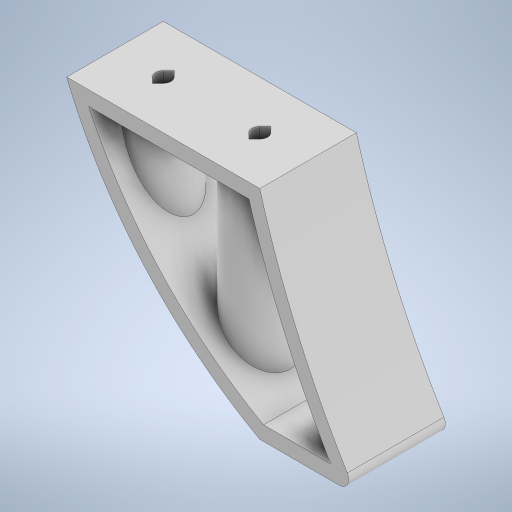
# Autodesk Inventor part: Feet
Saved by Autodesk Inventor 2023.1 (Build 271208000, 208)
## iProperties
Created: 2022-11-07
Part Number: Feet
Material: Generic
Document SubType Name: Modeling
Designer: nicol
Density: 1 g/cm^3
Appearance: Default
Author: nicol
Autodesk Inventor part; units mm, degrees
ref_plane "YZ Plane" through (0, 0, 0) normal (1, 0, 0) x (0, 1, 0)
ref_plane "XZ Plane" through (0, 0, 0) normal (0, 1, 0) x (-1, 0, 0)
ref_plane "XY Plane" through (0, 0, 0) normal (0, 0, 1) x (1, 0, 0)
sketch "Sketch1" plane through (0, 0, 0) normal (0, 0, 1) x (1, 0, 0)
  line L0 (0, 0) -> (20, 0)
  line L1 (-40, 45) -> (0, 45)
  arc A0 (-40, 45) -> (0, 0) centre (43.3923, 78.8487) ccw
  arc A1 (0, 45) -> (20, 0) centre (163.6669, 90.7964) ccw
  line L2 (0, 45) -> (0, 29.5126) construction
  line L3 (-40, 45) -> (-40, 23.133) construction
  dimension "d0" = 45
  dimension "d1" = 20
  dimension "d2" = 40
  dimension "d3" = 90
  constraints: 8 end point, 4 point on circle, 2 centre point, 2 horizontal, 2 vertical, 1 vertical alignment
  measures "d0" distance between parallel lines of L0 L1
  measures "d1" distance of L0.start L0.end
  measures "d2" distance of L1.start L1.end
  measures "d3" radius of A0
extrude "Extrusion1" add sketch "Sketch1" along normal blind 20
ref_plane "Work Plane1" through (-40, 40, 0) normal (0, 1, 0) x (1, 0, 0)
sketch "Sketch2" plane through (-40, 45, 0) normal (0, 1, 0) x (1, 0, 0)
  line L0 (40, 0) -> (40, -20) projected
  line L1 (0, 0) -> (0, -20) projected
  circle A0 centre (10, -10) radius 3.25
  circle A1 centre (30, -10) radius 3.25
  point P0 (0, -10)
  dimension "d7" = 10
  dimension "d8" = 10
  dimension "d9" = 6.5
  dimension "d10" = 6.5
  constraints: 2 centre point, 2 coincident, 2 horizontal alignment, 1 midpoint
  measures "d7" distance from line of L0 point (30, -10)
  measures "d8" distance from line of L1 point (10, -10)
  measures "d9" diameter of A0
  measures "d10" diameter of A1
hole "Hole1" at (-30, 45, 10) at (-10, 45, 10) direction (0, -1, 0) diameter 3.2 end through all
extrude "Extrusion2" cut sketch "Sketch2" against normal blind 58.25 from surface at -5
shell "Shell1" thickness 3 removed faces 2 at (-7.5312, 32.7187, 20) at (-7.5312, 32.7187, 0)
fillet "Fillet2" radius 2 1 edges at (20, 0, 10)
sketch "Sketch3" plane through (-40, 45, 0) normal (0, 1, 0) x (1, 0, 0)
  circle A0 centre (10, -10) radius 1.6 projected
  line L0 (40, 0) -> (0, 0) projected
  line L1 (0, 0) -> (0, -20) projected
  line L2 (40, -20) -> (0, -20) projected
  line L3 (40, 0) -> (40, -20) projected
  circle A1 centre (30, -10) radius 1.6 projected
  line L4 (30, -12.2627) -> (27.7373, -10)
  line L5 (27.7373, -10) -> (30, -7.7373)
  line L6 (30, -7.7373) -> (32.2627, -10)
  line L7 (32.2627, -10) -> (30, -12.2627)
  line L8 (30, -12.2627) -> (30, -7.7373) construction
  line L9 (27.7373, -10) -> (32.2627, -10) construction
  line L10 (10, -12.2627) -> (7.7373, -10)
  line L11 (7.7373, -10) -> (10, -7.7373)
  line L12 (10, -7.7373) -> (12.2627, -10)
  line L13 (12.2627, -10) -> (10, -12.2627)
  line L14 (10, -12.2627) -> (10, -7.7373) construction
  line L15 (7.7373, -10) -> (12.2627, -10) construction
  circle A2 centre (30, -10) radius 1.6 projected
  circle A3 centre (10, -10) radius 1.6 projected
  point P0 (11.1314, -8.8686)
  point P1 (8.8686, -8.8686)
  point P2 (11.1314, -11.1314)
  point P3 (8.8686, -11.1314)
  point P4 (31.1314, -11.1314)
  point P5 (28.8686, -11.1314)
  point P6 (31.1314, -8.8686)
  point P7 (28.8686, -8.8686)
  constraints: 24 end point, 4 midpoint, 4 parallel, 4 tangent, 2 perpendicular, 2 vertical
extrude "Extrusion3" cut sketch "Sketch3" against normal through all contours A0 L11 L12 | L13 L10 A0 | A1 L5 L6 | L7 L4 A1
body "Solid1"
